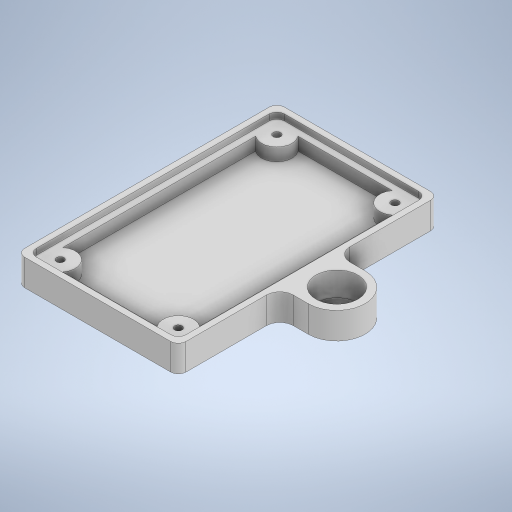
# Autodesk Inventor part: Thermister_Amp_Mount
Saved by Autodesk Inventor 2023 (Build 270158000, 158)
## iProperties
Created: 2022-05-20
Part Number: Thermister_Amp_Mount
Material: Generic
Document SubType Name: Modeling
Designer: devon
Density: 1 g/cm^3
Appearance: Default
Author: devon
Autodesk Inventor part; units mm, degrees
ref_plane "YZ Plane" through (0, 0, 0) normal (1, 0, 0) x (0, 1, 0)
ref_plane "XZ Plane" through (0, 0, 0) normal (0, 1, 0) x (-1, 0, 0)
ref_plane "XY Plane" through (0, 0, 0) normal (0, 0, 1) x (1, 0, 0)
sketch "Sketch1" plane through (0, 0, 0) normal (0, 1, 0) x (-1, 0, 0)
  line L0 (21.3, 34.3) -> (-21.3, 34.3)
  line L1 (-21.3, 34.3) -> (-21.3, -34.3)
  line L2 (-21.3, -34.3) -> (21.3, -34.3)
  line L3 (21.3, -34.3) -> (21.3, 34.3)
  line L4 (21.3, 34.3) -> (-21.3, -34.3) construction
  line L5 (-21.3, 34.3) -> (21.3, -34.3) construction
  point P0 (0, 0)
  dimension "d0" = 42.6
  dimension "d1" = 68.6
  constraints: 12 end point, 2 midpoint, 2 parallel, 1 horizontal, 1 perpendicular
  measures "d0" distance of L1.end L2.end
  measures "d1" distance of L0.end L1.end
extrude "Extrusion1" add sketch "Sketch1" along normal blind 7
sketch "Sketch2" plane through (0, 7, 0) normal (0, 1, 0) x (1, 0, 0)
  line L0 (-19.75, -32.75) -> (19.75, -32.75)
  line L1 (19.75, -32.75) -> (19.75, 32.75)
  line L2 (19.75, 32.75) -> (-19.75, 32.75)
  line L3 (-19.75, 32.75) -> (-19.75, -32.75)
  line L4 (-19.75, -32.75) -> (19.75, 32.75) construction
  line L5 (19.75, -32.75) -> (-19.75, 32.75) construction
  point P0 (0, 0)
  dimension "d4" = 39.5
  dimension "d5" = 65.5
  constraints: 12 end point, 2 midpoint, 2 parallel, 1 horizontal, 1 perpendicular
  measures "d4" distance of L1.end L2.end
  measures "d5" distance of L0.end L1.end
extrude "Extrusion2" cut sketch "Sketch2" against normal blind 1.6
sketch "Sketch3" plane through (0, 5.4, 0) normal (0, 1, 0) x (1, 0, 0)
  line L0 (-18.05, -31.05) -> (18.05, -31.05)
  line L1 (18.05, -31.05) -> (18.05, 31.05)
  line L2 (18.05, 31.05) -> (-18.05, 31.05)
  line L3 (-18.05, 31.05) -> (-18.05, -31.05)
  line L4 (-18.05, -31.05) -> (18.05, 31.05) construction
  line L5 (18.05, -31.05) -> (-18.05, 31.05) construction
  point P0 (0, 0)
  dimension "d8" = 36.1
  dimension "d9" = 62.1
  constraints: 12 end point, 2 midpoint, 2 parallel, 1 horizontal, 1 perpendicular
  measures "d8" distance of L1.end L2.end
  measures "d9" distance of L0.end L1.end
extrude "Extrusion3" cut sketch "Sketch3" against normal blind 3.4
sketch "Sketch4" plane through (0, 2, 0) normal (0, 1, 0) x (1, 0, 0)
  circle A0 centre (-15.6, 28.6) radius 4
  circle A1 centre (15.6, 28.6) radius 4
  circle A2 centre (-15.6, -28.6) radius 4
  circle A3 centre (15.6, -28.6) radius 4
  line L0 (-18.05, 31.05) -> (18.05, 31.05) projected
  line L1 (-18.05, -31.05) -> (-18.05, 31.05) projected
  point P0 (0, 0)
  dimension "d12" = 31.2
  dimension "d13" = 31.2
  dimension "d14" = 57.2
  dimension "d15" = 57.2
  dimension "d16" = 8
  dimension "d17" = 8
  dimension "d18" = 8
  dimension "d19" = 8
  dimension "d22" = 0
  dimension "d23" = 15.6
  dimension "d24" = 28.6
  dimension "d25" = 0
  constraints: 4 centre point
  measures "d12" distance of A1.centre A0.centre
  measures "d13" distance of A3.centre A2.centre
  measures "d14" distance of A3.centre A1.centre
  measures "d15" distance of A2.centre A0.centre
  measures "d16" diameter of A0
  measures "d17" diameter of A1
  measures "d18" diameter of A3
  measures "d19" diameter of A2
  measures "d22" vertical distance of A0.centre A1.centre
  measures "d23" horizontal distance of point (0, 0) A0.centre
  measures "d24" vertical distance of point (0, 0) A0.centre
  measures "d25" horizontal distance of A3.centre A1.centre
extrude "Extrusion4" add sketch "Sketch4" along normal blind 3.4
sketch "Sketch5" plane through (-15.6, 5.4, -28.6) normal (0, 1, 0) x (0.7071068, 0, -0.7071068)
  arc A0 (-3.9682, -0.5034) -> (3.9682, -0.5034) centre (0, 0) ccw projected
  circle A1 centre (0, 0) radius 1
  arc A2 (21.5584, -18.0935) -> (21.5584, -26.0299) centre (22.0617, -22.0617) ccw projected
  circle A3 centre (22.0617, -22.0617) radius 1
  arc A4 (-14.4166, -62.0049) -> (-22.353, -62.0049) centre (-18.3848, -62.5082) ccw projected
  circle A5 centre (-18.3848, -62.5082) radius 1
  arc A6 (-39.9431, -44.4147) -> (-39.9431, -36.4783) centre (-40.4465, -40.4465) ccw projected
  circle A7 centre (-40.4465, -40.4465) radius 1
  point P0 (-9.1924, -31.2541)
  point P1 (-0.6856, -2.9206)
  point P2 (0.6856, -2.9206)
  point P3 (-24.8409, 22.606)
  point P4 (-24.8409, 21.2347)
  point P5 (19.0704, 65.146)
  point P6 (17.6991, 65.146)
  dimension "d28" = 2
  dimension "d29" = 2
  dimension "d30" = 2
  dimension "d31" = 2
  constraints: 4 centre point, 4 coincident
  measures "d28" diameter of A1
  measures "d29" diameter of A3
  measures "d30" diameter of A5
  measures "d31" diameter of A7
extrude "Extrusion5" cut sketch "Sketch5" against normal blind 3.6
fillet "Fillet3" radius 2 8 edges at (-19.75, 6.2, -32.75) (19.75, 6.2, -32.75) (-19.75, 6.2, 32.75) (19.75, 6.2, 32.75) (-21.3, 3.5, -34.3) (-21.3, 3.5, 34.3) (21.3, 3.5, 34.3) (21.3, 3.5, -34.3)
sketch "Sketch8" plane through (21.3, 0, 32.3) normal (1, 0, 0) x (0, 0, -1)
  line L0 (63.05, 7) -> (1.55, 7) projected
  line L1 (0, 0) -> (64.6, 0) projected
  line L2 (39.8, 7) -> (24.8, 7)
  line L3 (24.8, 7) -> (24.8, 0)
  line L4 (24.8, 0) -> (39.8, 0)
  line L5 (39.8, 0) -> (39.8, 7)
  point P0 (32.3, 0)
  point P1 (39.8, 0)
  point P2 (24.8, 7)
  dimension "d49" = 15
  dimension "d50" = 7.5
  constraints: 8 end point, 2 parallel, 2 point on line, 1 horizontal, 1 perpendicular
  measures "d49" distance between parallel lines of L3 L5
  measures "d50" distance from line of point (32.3, 0) L5
extrude "Extrusion7" add sketch "Sketch8" along normal blind 15
sketch "Sketch9" plane through (0, 7, 0) normal (0, 1, 0) x (1, 0, 0)
  line L0 (36.3, 7.5) -> (36.3, -7.5) projected
  point P0 (0, 0)
  point P1 (28.8, 0.0728)
  dimension "d60" = 7.5
  measures "d60" distance from line of L0 point (28.8, 0.073)
hole "Hole2" at (28.8, 7, -0.0728) direction (0, -1, 0) diameter 6.756 end through all counterbore diameter 11.113 counterbore depth 6.35 clearance for "Socket Head Cap Screw" size "1/4" standard "Ansi Unified Screw Threads"
fillet "Fillet4" radius 3.5 2 edges at (21.3, 3.5, -7.5) (21.3, 3.5, 7.5)
fillet "Fillet5" radius 7.5 2 edges at (36.3, 3.5, 7.5) (36.3, 3.5, -7.5)
equation "\"d13\" = d12"
equation "\"d14\" = d15"
equation "\"d23\" = 0.5 * d12"
equation "\"d24\" = 0.5 * d15"
equation "\"d50\" = 0.5 * d49"
body "Solid1"
